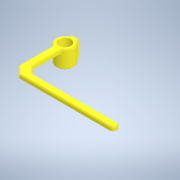
# Autodesk Inventor part: wing_lock
Saved by Autodesk Inventor 2021 (Build 250183000, 183)
## iProperties
Created: 2021-02-04
Part Number: wing_lock
Material: Generic
Document SubType Name: Modeling
Designer: Daniel
Density: 1 g/cm^3
Appearance: Default
Author: Daniel
Autodesk Inventor part; units mm, degrees
ref_plane "YZ Plane" through (0, 0, 0) normal (1, 0, 0) x (0, 1, 0)
ref_plane "XZ Plane" through (0, 0, 0) normal (0, 1, 0) x (-1, 0, 0)
ref_plane "XY Plane" through (0, 0, 0) normal (0, 0, 1) x (1, 0, 0)
sketch "Sketch1" plane through (0, 0, 0) normal (0, 1, 0) x (-1, 0, 0)
  arc A0 (-3.999679, -49.949292) -> (4, -50) centre (0, -50) ccw
  line L0 (0, 0) -> (-102, 0) construction
  line L1 (-3.999679, -4) -> (-102, -4)
  line L2 (-102, 4) -> (4, 4)
  arc A1 (-102, 4) -> (-102, -4) centre (-102, 0) ccw
  circle A2 centre (0, -50) radius 2.25
  line L3 (4, -50) -> (4, 4)
  circle A3 centre (0, -50) radius 6.375
  circle A4 centre (0, -50) radius 9.375
  line L4 (-85.872983, 1) -> (-105.872983, 1)
  line L5 (-105.872983, -1) -> (-85.872983, -1)
  line L6 (-85.872983, -1) -> (-85.872983, 1)
  line L7 (-3.999679, -49.949292) -> (-3.999679, -4)
  line L8 (-4, -58.478834) -> (4, -58.478834)
  line L9 (4, -58.478834) -> (4, -61.375)
  line L10 (4, -61.375) -> (-4, -61.375)
  line L11 (-4, -61.375) -> (-4, -58.478834)
  circle A5 centre (0, -50) radius 11.375 construction
  line L12 (-11.070746, -4) -> (-3.999679, -11.071068)
  line L13 (-4.928611, 4) -> (4, -4.928611)
  point P0 (-51, 0)
  point P1 (-8.518949, -5)
  point P2 (4, -41.521166)
  point P3 (-92.743026, 0)
  point P4 (-3.999679, -41.521014)
  point P5 (4, -45.036068)
  point P6 (-3.999679, -45.035809)
  dimension "d9" = 4.5
  dimension "d24" = 4
  dimension "d29" = 12.75
  dimension "d30" = 3
  dimension "d46" = 102
  dimension "d48" = 2
  dimension "d49" = 20
  dimension "d50" = 1
  dimension "d52" = 50
  dimension "d53" = 7.99968
  dimension "d54" = 8
  dimension "d55" = 90
  dimension "d56" = 8
  dimension "d58" = 5
  dimension "d59" = 10
  dimension "d60" = 5
  dimension "d61" = 45
  constraints: 30 end point, 9 parallel, 8 point on circle, 6 centre point, 5 coincident, 5 point on line, 4 tangent, 2 perpendicular, 1 horizontal, 1 midpoint, 1 vertical alignment
  measures "d9" diameter of A2
  measures "d24" radius of A0
  measures "d29" diameter of A3
  measures "d30" radial gap between concentric circles of A4 A3
  measures "d46" distance of L0.start L0.end
  measures "d48" distance between parallel lines of L4 L5
  measures "d49" distance of L4.start L4.end
  measures "d50" distance between parallel lines of L0 L4
  measures "d52" distance of A0.centre point (0, 0)
  measures "d53" distance between parallel lines of L7 L3
  measures "d54" distance between parallel lines of L1 L2
  measures "d55" angle of L1 L7
  measures "d56" distance of L8.start L8.end
  measures "d58" radial gap between concentric circles of A3 A5
  measures "d59" distance between parallel lines of L13 L12
  measures "d60" distance from line of L1.start L12
  measures "d61" angle of L1 L12
extrude "Extrusion1" add sketch "Sketch1" along normal blind 4 contours L7 A4 L3 A3 | A3 L3 A4 L8 L7 | L7 L1 A1 L5 L6 L4 L2 L13 L3 A4 | L8 A4 | A4 L9 L10 L11 | L12 L1 L7 | A1 L4 L6 L5
sketch "Sketch7" plane through (0, 0, 0) normal (0, -1, 0) x (1, 0, 0)
  arc A0 (-4, -41.521166) -> (3.999679, -41.521014) centre (0, -50) ccw
  circle A1 centre (0, -50) radius 6.4
  circle A2 centre (0, -50) radius 9.375
  line L0 (4.928611, 4) -> (102, 4)
  arc A3 (102, -4) -> (102, 4) centre (102, 0) ccw
  line L1 (102, -4) -> (11.070746, -4)
  arc A4 (4, -58.478834) -> (3.999679, -41.521014) centre (0, -50) ccw
  line L2 (4, -58.478834) -> (4, -61.375)
  line L3 (4, -61.375) -> (-4, -61.375)
  line L4 (-4, -61.375) -> (-4, -58.478834)
  arc A5 (-4, -41.521166) -> (-4, -58.478834) centre (0, -50) ccw
  circle A6 centre (0, -50) radius 6.375
  line L5 (11.070746, -4) -> (3.999679, -11.071068)
  line L6 (3.999679, -11.071068) -> (3.999679, -41.521014)
  line L7 (-4, -41.521166) -> (-4, -4.928611)
  line L8 (-4, -4.928611) -> (4.928611, 4)
  point P0 (0, 0)
  point P1 (3.999679, -41.521014)
  point P2 (-4, -58.478834)
  dimension "d31" = 12.8
  constraints: 2 centre point, 2 coincident, 1 concentric
  measures "d31" diameter of A1
extrude "Extrusion6" add sketch "Sketch7" along normal blind 15 contours A2 A0 | A0 L2 L3 L4
sketch "Sketch8" plane through (8.451183, 0, -61.375) normal (0, 0, 1) x (1, 0, 0)
  circle A0 centre (-8.451183, -7) radius 1.65
  line L0 (-17.826183, -15) -> (0.923817, -15)
  point P0 (-8.451183, 0)
  point P1 (-2.689333, 8)
  point P2 (-8.451183, -15)
  point P3 (-8.451183, -15)
  dimension "d34" = 3.3
  dimension "d47" = 8
  constraints: 2 vertical alignment, 1 centre point, 1 midpoint
  measures "d34" diameter of A0
  measures "d47" distance from line of L0 A0.centre
extrude "Extrusion7" cut sketch "Sketch8" along normal up to surface round surface about axis through (0, 0, -50) along (0, 1, 0) radius 6.375 far side no
fillet "Fillet2" radius 2 3 edges at (-0.0002, 0, -40.625) (-4, 2, -41.5212) (3.9997, 2, -41.521)
chamfer "Chamfer1" distance 1 angle 45 14 edges at (-9.3596, 4, -50.5379) (-4.2522, 4, -41.3083) (-4, 4, -22.6324) (9.3596, 4, -50.5378) (4.2519, 4, -41.3081) (3.9997, 4, -25.7035) (53.4643, 4, 4) (106, 4, 0) (56.5354, 4, -4) (4, 4, -59.9269) (-4, 4, -59.9269) (0, 4, -61.375) (7.5352, 4, -7.5355) (0.4643, 4, -0.4643)
chamfer "Chamfer2" distance 1 angle 45 5 edges at (-6.4, -15, -50) (0, -15, -40.625) (4, -15, -59.9269) (0, -15, -61.375) (-4, -15, -59.9269)
equation "\"d50\" = 0.5 * d48"
body "Solid1"
